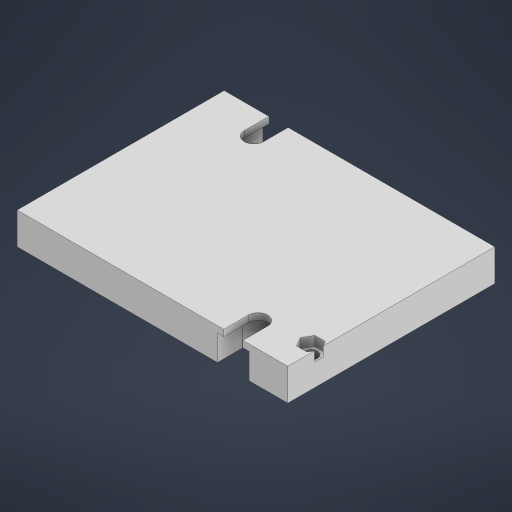
# Autodesk Inventor part: base_fuentePoder_12v5a
Saved by Autodesk Inventor 2023 (Build 270158000, 158)
## iProperties
Created: 2023-03-01
Part Number: base_fuentePoder_12v5a
Material: Generic
Document SubType Name: Modeling
Designer: tomas
Density: 1 g/cm^3
Appearance: Default
Author: tomas
## iProperties of the stored document base_fuentePoder_12v5a_3DPrint.ipt
Created: 2023-03-01
Part Number: base_fuentePoder_12v5a_3DPrint
Material: Generic
Document SubType Name: Modeling
Designer: tomas
Density: 1 g/cm^3
Appearance: Default
Author: tomas
Autodesk Inventor part; units mm, degrees
ref_plane "YZ Plane" through (0, 0, 0) normal (1, 0, 0) x (0, 1, 0)
ref_plane "XZ Plane" through (0, 0, 0) normal (0, 1, 0) x (-1, 0, 0)
ref_plane "XY Plane" through (0, 0, 0) normal (0, 0, 1) x (1, 0, 0)
sketch "Sketch1" plane through (0, 0, 0) normal (0, 1, 0) x (-1, 0, 0)
  line L0 (42.5, -32.5) -> (42.5, 32.5)
  line L1 (-42.5, 32.5) -> (-42.5, -32.5)
  line L2 (-42.5, -32.5) -> (42.5, 32.5) construction
  line L3 (42.5, -32.5) -> (-42.5, 32.5) construction
  line L4 (-25.4, -24.765) -> (25.4, -24.765) construction
  line L5 (25.4, -24.765) -> (25.4, 24.765) construction
  line L6 (25.4, 24.765) -> (-25.4, 24.765) construction
  line L7 (-25.4, 24.765) -> (-25.4, -24.765) construction
  line L8 (-25.4, -24.765) -> (25.4, 24.765) construction
  line L9 (25.4, -24.765) -> (-25.4, 24.765) construction
  arc A0 (-28.4, 24.765) -> (-22.4, 24.765) centre (-25.4, 24.765) ccw
  arc A1 (-30.4, 24.765) -> (-20.4, 24.765) centre (-25.4, 24.765) ccw
  arc A2 (28.4, -24.765) -> (22.4, -24.765) centre (25.4, -24.765) ccw
  arc A3 (30.4, -24.765) -> (20.4, -24.765) centre (25.4, -24.765) ccw
  line L10 (-20.4, 32.5) -> (-20.4, 24.765)
  line L11 (-30.4, 32.5) -> (-30.4, 24.765)
  line L12 (-28.4, 32.5) -> (-28.4, 24.765)
  line L13 (-22.4, 32.5) -> (-22.4, 24.765)
  line L14 (30.4, -24.765) -> (30.4, -32.5)
  line L15 (28.4, -24.765) -> (28.4, -32.5)
  line L16 (22.4, -24.765) -> (22.4, -32.5)
  line L17 (20.4, -24.765) -> (20.4, -32.5)
  line L18 (-42.5, -32.5) -> (22.4, -32.5)
  line L19 (28.4, -32.5) -> (42.5, -32.5)
  line L20 (42.5, 32.5) -> (-22.4, 32.5)
  line L21 (-28.4, 32.5) -> (-42.5, 32.5)
  point P0 (0, 0)
  dimension "d2" = 50.8
  dimension "d3" = 49.53
  dimension "d4" = 6
  dimension "d5" = 10
  constraints: 44 end point, 11 perpendicular, 9 parallel, 8 point on circle, 6 point on line, 4 centre point, 4 coincident, 4 midpoint, 4 tangent, 3 horizontal, 2 equal radius
  measures "d2" distance of L6.end L5.end
  measures "d3" distance of L5.end L4.end
  measures "d4" diameter of A0
  measures "d5" diameter of A1
sketch "Sketch2" plane through (0, 0, 0) normal (0, 1, 0) x (-1, 0, 0)
  line L0 (-43, -29.25) -> (43, -29.25)
  line L1 (43, -29.25) -> (43, 29.25)
  line L2 (43, 29.25) -> (-43, 29.25)
  line L3 (-43, 29.25) -> (-43, -29.25)
  line L4 (-43, -29.25) -> (43, 29.25) construction
  line L5 (43, -29.25) -> (-43, 29.25) construction
  circle A0 centre (39.6, -24.85) radius 1.4
  line L6 (41, -24.85) -> (39.6, -24.85)
  line L7 (39.6, -24.85) -> (39.6, -26.25)
  circle A1 centre (-40, 22.75) radius 2
  line L8 (-38, 22.75) -> (-43, 22.75) construction
  line L9 (-40, 24.75) -> (-40, 29.25) construction
  line L10 (-40, 24.75) -> (-40, 22.75) construction
  point P0 (0, 0)
  dimension "d6" = 86
  dimension "d7" = 58.5
  dimension "d8" = 2.8
  dimension "d9" = 3
  dimension "d10" = 2
  dimension "d11" = 4
  dimension "d12" = 5
  dimension "d13" = 4.5
  constraints: 22 end point, 4 perpendicular, 4 point on circle, 2 centre point, 2 horizontal, 2 midpoint, 2 parallel, 2 point on line, 1 vertical
  measures "d6" distance of L2.end L1.end
  measures "d7" distance of L1.end L0.end
  measures "d8" diameter of A0
  measures "d9" distance from line of L0 L7.end
  measures "d10" distance from line of L1 L6.start
  measures "d11" diameter of A1
  measures "d12" distance of L8.start L8.end
  measures "d13" distance of L9.start L9.end
extrude "Extrusion1" add sketch "Sketch1" along normal blind 10
extrude "Extrusion2" cut sketch "Sketch1" along normal blind 8 contours L19 L15 A2 L16 L18 L17 A3 L14 | L10 A1 L11 L21 L12 A0 L13 L20
extrude "Extrusion3" add sketch "Sketch2" against normal blind 5 contours L6 L7 A0 | A0 L7 L6
extrude "Extrusion4" cut sketch "Sketch2" along normal through all contours A1
sketch "Sketch3" plane through (0, 10, 0) normal (0, 1, 0) x (1, 0, 0)
  circle A0 centre (40, -22.75) radius 2 projected
  arc A1 (-28.4, 24.765) -> (-22.4, 24.765) centre (-25.4, 24.765) ccw projected
  line L0 (-28.4, 24.765) -> (-28.4, 32.5) projected
  line L1 (-28.4, 32.5) -> (-42.5, 32.5) projected
  line L2 (-42.5, 32.5) -> (-42.5, -32.5) projected
  line L3 (-42.5, -32.5) -> (22.4, -32.5) projected
  line L4 (22.4, -32.5) -> (22.4, -24.765) projected
  arc A2 (28.4, -24.765) -> (22.4, -24.765) centre (25.4, -24.765) ccw projected
  line L5 (28.4, -24.765) -> (28.4, -32.5) projected
  line L6 (28.4, -32.5) -> (42.5, -32.5) projected
  line L7 (42.5, -32.5) -> (42.5, 32.5) projected
  line L8 (42.5, 32.5) -> (-22.4, 32.5) projected
  line L9 (-22.4, 32.5) -> (-22.4, 24.765) projected
  circle A3 centre (40, -22.75) radius 2.85
  line L10 (41.6454, -19.9) -> (43.2909, -22.75)
  line L11 (43.2909, -22.75) -> (41.6454, -25.6)
  line L12 (41.6454, -25.6) -> (38.3546, -25.6)
  line L13 (38.3546, -25.6) -> (36.7091, -22.75)
  line L14 (36.7091, -22.75) -> (38.3546, -19.9)
  line L15 (38.3546, -19.9) -> (41.6454, -19.9)
  point P0 (0, 0)
  point P1 (40, -19.9)
  dimension "d22" = 5.7
  constraints: 12 end point, 2 coincident, 1 midpoint, 1 vertical alignment, 15 other
extrude "Extrusion5" cut sketch "Sketch3" against normal blind 3 contours A0 | A3 L7 | L10 L11 A3 | L7 A3 | A3 L15 L10 | L11 L12 A3 | A3 L14 L15 | L12 L13 A3 | A3 L13 L14
body "Solid1"
